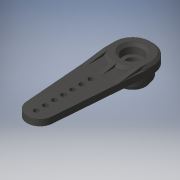
# Autodesk Inventor part: ser Horn
Saved by Autodesk Inventor 2016 (Build 200138000, 138)
## iProperties
Created: 2017-02-10
Part Number: ser Horn
Material: PC/ABS Plastic
Document SubType Name: Modeling
Designer: Nanjar
Density: 0.357273 g/cm^3
Appearance: Smooth - White
Author: Nanjar
Autodesk Inventor part; units mm, degrees
note: some values were not read from the file. Chosen so that the rebuilt part matches the saved one: edges of "Chamfer8".
ref_plane "YZ Plane" through (0, 0, 0) normal (1, 0, 0) x (0, 1, 0)
ref_plane "XZ Plane" through (0, 0, 0) normal (0, 1, 0) x (-1, 0, 0)
ref_plane "XY Plane" through (0, 0, 0) normal (0, 0, 1) x (1, 0, 0)
sketch "Sketch3" plane through (0, 0, 0) normal (0, 1, 0) x (-1, 0, 0)
  circle A0 centre (0, 0) radius 5.25
  circle A1 centre (0, 0) radius 2.025
  dimension "d8" = 10.5
  dimension "d9" = 4.05
  constraints: 2 centre point, 2 coincident
  measures "d8" diameter of A0
  measures "d9" diameter of A1
extrude "Extrusion2" add sketch "Sketch3" along normal blind 7.9
sketch "Sketch5" plane through (0, 0, 0) normal (0, -1, 0) x (1, 0, 0)
  circle A0 centre (0, 0) radius 3.075
  dimension "d13" = 6.15
  constraints: 1 centre point, 1 coincident
  measures "d13" diameter of A0
extrude "Extrusion3" cut sketch "Sketch5" against normal blind 3.85
sketch "Sketch6" plane through (0, 7.9, 0) normal (0, 1, 0) x (1, 0, 0)
  circle A0 centre (0, 0) radius 3.25
  dimension "d16" = 6.5
  constraints: 1 centre point, 1 coincident
  measures "d16" diameter of A0
extrude "Extrusion4" cut sketch "Sketch6" against normal blind 3.05
chamfer "Chamfer1" distance 0.9 angle 45 1 edges at (-3.25, 7.9, 0)
chamfer "Chamfer2" distance 1.4 angle 35 1 edges at (5.25, 0, 0) measured on face at (-5.233, 5.2667, -0.4224)
sketch "Sketch7" plane through (0, 7.9, 0) normal (0, 1, 0) x (1, 0, 0)
  circle A0 centre (0, 0) radius 6.65
  circle A1 centre (0, 0) radius 4.05
  dimension "d25" = 13.3
  constraints: 2 centre point, 2 coincident
  measures "d25" diameter of A0
extrude "Extrusion5" add sketch "Sketch7" against normal blind 3.1
sketch "Sketch10" plane through (0, 4.8, 0) normal (0, -1, 0) x (1, 0, 0)
  line L0 (7.695, -6.65) -> (-7.0508, -6.65) construction
  circle A0 centre (0, 0) radius 6.65 construction
  line L1 (7.695, 34.7) -> (-9.9526, 34.7) construction
  arc A1 (4.2368, 30.785) -> (-4.2368, 30.785) centre (0, 30.45) ccw
  line L2 (0, 30.45) -> (0, 0) construction
  line L3 (4.2368, 30.785) -> (6.6293, 0.5241)
  line L4 (-4.2368, 30.785) -> (-6.6293, 0.5241)
  arc A2 (-6.6293, 0.5241) -> (6.6293, 0.5241) centre (0, 0) ccw
  circle A3 centre (0, 0) radius 4.05
  dimension "d33" = 41.35
  dimension "d34" = 8.5
  constraints: 10 end point, 6 tangent, 4 centre point, 4 point on circle, 2 coincident
  measures "d33" distance between parallel lines of L1 L0
  measures "d34" diameter of A1
extrude "Extrusion7" add sketch "Sketch10" against normal blind 2.1
sketch "Sketch11" plane through (0, 6.9, 0) normal (0, 1, 0) x (1, 0, 0)
  line L0 (-8.7036, -34.7) -> (5.9781, -34.7) construction
  arc A0 (-4.2368, -30.785) -> (4.2368, -30.785) centre (0, -30.45) ccw construction
  line L1 (-9.4118, -32.5) -> (5.9781, -32.5) construction
  circle A1 centre (0, -31.675) radius 0.825
  line L2 (-3.4465, -30.85) -> (3.2814, -30.85) construction
  line L3 (-3.1615, -29.5) -> (2.5188, -29.5) construction
  circle A2 centre (0, -28.675) radius 0.825
  line L4 (0, -34.7) -> (0, 0) construction
  circle A3 centre (0, -25.675) radius 0.825
  circle A4 centre (0, -22.675) radius 0.825
  circle A5 centre (0, -19.675) radius 0.825
  circle A6 centre (0, -16.675) radius 0.825
  circle A7 centre (0, -13.675) radius 0.825
  dimension "d40" = 2.2
  dimension "d41" = 1.65
  dimension "d42" = 1.35
  dimension "d43" = 1.65
  dimension "d44" = 3
  dimension "d47" = 3
  constraints: 10 end point, 7 centre point, 4 horizontal, 4 tangent, 2 vertical, 1 point on circle, 10 other
  measures "d40" distance between parallel lines of L0 L1
  measures "d41" diameter of A1
  measures "d42" distance between parallel lines of L3 L2
  measures "d43" diameter of A2
  measures "d44" distance of A1.centre A2.centre
  measures "d47" distance of A2.centre A3.centre
extrude "Extrusion8" cut sketch "Sketch11" against normal blind 2.1
sketch "Sketch12" plane through (0, 6.9, 0) normal (0, 1, 0) x (1, 0, 0)
  arc A0 (-5.8287, -1.8994) -> (-4.5287, -4.1319) centre (0, 0) ccw
  arc A1 (-0.65, -6.0958) -> (0.65, -6.0958) centre (0, 0) ccw
  line L0 (-5.8287, -1.8994) -> (-5.8287, -10.65)
  line L1 (-5.8287, -10.65) -> (-4.5287, -10.65)
  line L2 (-4.5287, -10.65) -> (-4.5287, -4.1319)
  line L3 (0.65, -10.65) -> (-0.65, -10.65)
  line L4 (-0.65, -10.65) -> (-0.65, -6.0958)
  line L5 (0.65, -10.65) -> (0.65, -6.0958)
  line L6 (0, -12.8402) -> (0, 0) construction
  arc A2 (4.5287, -4.1319) -> (5.8287, -1.8994) centre (0, 0) ccw
  line L7 (5.8287, -1.8994) -> (5.8287, -10.65)
  line L8 (5.8287, -10.65) -> (4.5287, -10.65)
  line L9 (4.5287, -10.65) -> (4.5287, -4.1319)
  constraints: 20 end point, 6 point on circle, 4 symmetric about line, 3 centre point, 3 perpendicular, 2 vertical, 1 horizontal, 1 parallel, 1 other
extrude "Extrusion9" add sketch "Sketch12" along normal blind 1
fillet "Fillet2" radius 0.5 1 edges at (5.25, 1.4, 0)
chamfer "Chamfer8" distance 0.82 angle 45 1 edges at (0, 7.9, -6.65)
fillet "Fillet4" radius 0.4 1 edges at (0, 7.08, -6.65)
chamfer "Chamfer9" distance 0.82 angle 45 2 edges at (-2.733, 7.9, 6.0625) (2.733, 7.9, 6.0625)
fillet "Fillet5" radius 0.4 2 edges at (2.733, 7.08, 6.0625) (-2.733, 7.08, 6.0625)
chamfer "Chamfer10" distance 6.978 distance2 1 1 edges at (-5.1787, 7.9, 10.65) measured on face at (5.3954, 7.9, 4.8145)
chamfer "Chamfer11" distance 4.856 distance2 1 1 edges at (0, 7.9, 10.65) measured on face at (5.3954, 7.9, 4.8145)
chamfer "Chamfer12" distance 6.978 distance2 1 1 edges at (5.1787, 7.9, 10.65) measured on face at (5.3954, 7.9, 4.8145)
body "Solid2"
